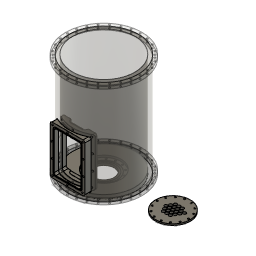
Smooth.SAQ.Pix.Vessel.5.9.2023. (Autodesk Fusion 360 design; units mm, degrees)
Autodesk Fusion 360 part; units mm, degrees
note: some values were not read from the file. Chosen so that the rebuilt part matches the saved one: which bodies a step acts on. Set by a fixed rule: which sketch regions a step uses.
sketch "Vessel.Base" plane through (0, 0, 0) normal (0, 1, 0) x (1, 0, 0)
  circle A0 centre (0, 0) radius 40
  circle A1 centre (0, 0) radius 30
  circle A2 centre (0, 0) radius 100
  circle A3 centre (0, 0) radius 110
  line L0 (0, 0) -> (105, 0) construction
  circle A4 centre (105, 0) radius 2.3
  circle A5 centre (102.3674, 23.3647) radius 2.3
  circle A6 centre (94.6017, 45.5578) radius 2.3
  circle A7 centre (82.0923, 65.4664) radius 2.3
  circle A8 centre (65.4664, 82.0923) radius 2.3
  circle A9 centre (45.5578, 94.6017) radius 2.3
  circle A10 centre (23.3647, 102.3674) radius 2.3
  circle A11 centre (0, 105) radius 2.3
  circle A12 centre (-23.3647, 102.3674) radius 2.3
  circle A13 centre (-45.5578, 94.6017) radius 2.3
  circle A14 centre (-65.4664, 82.0923) radius 2.3
  circle A15 centre (-82.0923, 65.4664) radius 2.3
  circle A16 centre (-94.6017, 45.5578) radius 2.3
  circle A17 centre (-102.3674, 23.3647) radius 2.3
  circle A18 centre (-105, 0) radius 2.3
  circle A19 centre (-102.3674, -23.3647) radius 2.3
  circle A20 centre (-94.6017, -45.5578) radius 2.3
  circle A21 centre (-82.0923, -65.4664) radius 2.3
  circle A22 centre (-65.4664, -82.0923) radius 2.3
  circle A23 centre (-45.5578, -94.6017) radius 2.3
  circle A24 centre (-23.3647, -102.3674) radius 2.3
  circle A25 centre (0, -105) radius 2.3
  circle A26 centre (23.3647, -102.3674) radius 2.3
  circle A27 centre (45.5578, -94.6017) radius 2.3
  circle A28 centre (65.4664, -82.0923) radius 2.3
  circle A29 centre (82.0923, -65.4664) radius 2.3
  circle A30 centre (94.6017, -45.5578) radius 2.3
  circle A31 centre (102.3674, -23.3647) radius 2.3
  circle A32 centre (0, 0) radius 90
  circle A33 centre (0, 0) radius 50
  line L1 (0, 0) -> (45, 0) construction
  circle A34 centre (45, 0) radius 2.3
  circle A35 centre (40.5436, 19.5248) radius 2.3
  circle A36 centre (28.057, 35.1824) radius 2.3
  circle A37 centre (10.0134, 43.8718) radius 2.3
  circle A38 centre (-10.0134, 43.8718) radius 2.3
  circle A39 centre (-28.057, 35.1824) radius 2.3
  circle A40 centre (-40.5436, 19.5248) radius 2.3
  circle A41 centre (-45, 0) radius 2.3
  circle A42 centre (-40.5436, -19.5248) radius 2.3
  circle A43 centre (-28.057, -35.1824) radius 2.3
  circle A44 centre (-10.0134, -43.8718) radius 2.3
  circle A45 centre (10.0134, -43.8718) radius 2.3
  circle A46 centre (28.057, -35.1824) radius 2.3
  circle A47 centre (40.5436, -19.5248) radius 2.3
  circle A48 centre (0, 0) radius 35
  line L2 (0, 0) -> (0, -105) construction
  line L3 (0, 0) -> (0, -95) construction
  dimension "d1" = 80
  dimension "d2" = 60
  dimension "d3" = 200
  dimension "d4" = 220
  dimension "d5" = 4.6
  dimension "d7" = 360
  dimension "d10" = 180
  dimension "d85" = 100
  dimension "d105" = 45
  dimension "d106" = 4.6
  dimension "d108" = 360
  dimension "d111" = 70
  dimension "d187" = 105
  dimension "d188" = 95
  constraint coincident A0.centre A1.centre
  constraint concentric A1 A2
  constraint concentric A2 A3
  constraint horizontal L0
  constraint coincident L0.end A4.centre
  constraint concentric A0 A33
  constraint horizontal L1
  constraint coincident L1.end A34.centre
  constraint concentric A33 A48
  constraint vertical L2
  constraint parallel L2 L3
  measures "d1" diameter of A0
  measures "d2" diameter of A1
  measures "d3" diameter of A2
  measures "d4" diameter of A3
  measures "d5" diameter of A4
  measures "d10" diameter of A32
  measures "d85" diameter of A33
  measures "d105" distance of A0.centre L1.end
  measures "d106" diameter of A34
  measures "d111" diameter of A48
  measures "d187" distance of A0.centre A25.centre
  measures "d188" distance of A0.centre L3.end
extrude "Extrude1" add sketch "Vessel.Base" along normal blind 10 contours A3 makes body 1
extrude "Extrude2" add sketch "Vessel.Base" along normal blind 300 separate body contours A2 makes body 2
extrude "Extrude3" add 1 faces at (-98.8073, 10, -35.1548) along direction (0, 1, 0) blind 10 separate body on bodies 1 makes body 3
move_body "Move1" bodies 3 to x (1, 0, 0) y (0, 1, 0) z (0, 0, 1) at (0, 280, 0)
extrude "Extrude5" add sketch "Vessel.Base" along normal blind 10 separate body contours A0 | A48 makes body 4
extrude "Extrude6" add sketch "Vessel.Base" along normal blind 11.6 contours A32 | A33 | A34 | A35 | A36 | A37 | A38 | A39 | A40 | A41 | A42 | A43 | A44 | A45 | A46 | A47 bodies 4
extrude "Extrude7" cut 1 faces at (36.4061, 10, 3.4777) along direction (0, -1, 0) blind 1.6 on bodies 4 bodies 4
sketch "Readout-Holder" plane through (0, 0, 0) normal (0, 1, 0) x (1, 0, 0)
  circle A0 centre (200, 0) radius 30
  circle A1 centre (200, 0) radius 1 construction
  circle A2 centre (210, 0) radius 1 construction
  circle A3 centre (220, 0) radius 1 construction
  circle A4 centre (180, 0) radius 1 construction
  circle A5 centre (205, 8.6603) radius 1 construction
  circle A6 centre (195, 8.6603) radius 1 construction
  circle A7 centre (190, 0) radius 1 construction
  circle A8 centre (195, -8.6603) radius 1 construction
  circle A9 centre (205, -8.6603) radius 1 construction
  circle A10 centre (210, 17.3205) radius 1 construction
  circle A11 centre (190, 17.3205) radius 1 construction
  circle A12 centre (180, 0) radius 1 construction
  circle A13 centre (190, -17.3205) radius 1 construction
  circle A14 centre (210, -17.3205) radius 1 construction
  circle A15 centre (200, 17.3205) radius 1 construction
  circle A16 centre (200, -17.3205) radius 1 construction
  circle A17 centre (185, 8.6603) radius 1 construction
  circle A18 centre (215, 8.6603) radius 1 construction
  circle A19 centre (185, -8.6603) radius 1 construction
  circle A20 centre (215, -8.6603) radius 1 construction
  circle A21 centre (200, 0) radius 40 construction
  circle A22 centre (200, 0) radius 4.5
  circle A23 centre (210, 0) radius 4.5
  circle A24 centre (220, 0) radius 4.5
  circle A25 centre (215, 8.6603) radius 4.5
  circle A26 centre (205, 8.6603) radius 4.5
  circle A27 centre (195, 8.6603) radius 4.5
  circle A28 centre (185, 8.6603) radius 4.5
  circle A29 centre (190, 17.3205) radius 4.5
  circle A30 centre (200, 17.3205) radius 4.5
  circle A31 centre (210, 17.3205) radius 4.5
  circle A32 centre (190, 0) radius 4.5
  circle A33 centre (180, 0) radius 4.5
  circle A34 centre (185, -8.6603) radius 4.5
  circle A35 centre (195, -8.6603) radius 4.5
  circle A36 centre (205, -8.6603) radius 4.5
  circle A37 centre (215, -8.6603) radius 4.5
  circle A38 centre (190, -17.3205) radius 4.5
  circle A39 centre (200, -17.3205) radius 4.5
  circle A40 centre (210, -17.3205) radius 4.5
  circle A41 centre (200, 0) radius 50
  line L0 (200, 0) -> (245, 0) construction
  circle A42 centre (245, 0) radius 2.3
  circle A43 centre (240.5436, 19.5248) radius 2.3
  circle A44 centre (228.057, 35.1824) radius 2.3
  circle A45 centre (210.0134, 43.8718) radius 2.3
  circle A46 centre (189.9866, 43.8718) radius 2.3
  circle A47 centre (171.943, 35.1824) radius 2.3
  circle A48 centre (159.4564, 19.5248) radius 2.3
  circle A49 centre (155, 0) radius 2.3
  circle A50 centre (159.4564, -19.5248) radius 2.3
  circle A51 centre (171.943, -35.1824) radius 2.3
  circle A52 centre (189.9866, -43.8718) radius 2.3
  circle A53 centre (210.0134, -43.8718) radius 2.3
  circle A54 centre (228.057, -35.1824) radius 2.3
  circle A55 centre (240.5436, -19.5248) radius 2.3
  line L1 (215, 8.6603) -> (225, 8.6603) construction
  circle A56 centre (225, 8.6603) radius 1 construction
  circle A57 centre (225, 8.6603) radius 4.5
  dimension "d23" = 60
  dimension "d25" = 2
  dimension "d28" = 20
  dimension "d29" = 0
  dimension "d32" = -20
  dimension "d33" = 0
  dimension "d35" = 360
  dimension "d37" = 360
  dimension "d39" = 2
  dimension "d41" = 2
  dimension "d46" = 2
  dimension "d47" = 2
  dimension "d48" = 2
  dimension "d49" = 2
  dimension "d52" = 80
  dimension "d63" = 9
  dimension "d64" = 9
  dimension "d65" = 9
  dimension "d66" = 9
  dimension "d67" = 9
  dimension "d68" = 9
  dimension "d69" = 9
  dimension "d70" = 9
  dimension "d71" = 9
  dimension "d72" = 9
  dimension "d73" = 9
  dimension "d74" = 9
  dimension "d75" = 9
  dimension "d76" = 9
  dimension "d77" = 9
  dimension "d78" = 9
  dimension "d79" = 9
  dimension "d80" = 9
  dimension "d100" = 4.6
  dimension "d102" = 360
  dimension "d117" = 10
  dimension "d118" = 2
  dimension "d119" = 9
  constraint concentric A0 A1
  constraint concentric A0 A21
  constraint concentric A1 A22
  constraint concentric A2 A23
  constraint concentric A3 A24
  constraint concentric A18 A25
  constraint concentric A5 A26
  constraint concentric A6 A27
  constraint concentric A17 A28
  constraint concentric A11 A29
  constraint concentric A15 A30
  constraint concentric A10 A31
  constraint concentric A7 A32
  constraint concentric A12 A33
  constraint concentric A19 A34
  constraint concentric A8 A35
  constraint concentric A9 A36
  constraint concentric A20 A37
  constraint concentric A13 A38
  constraint concentric A16 A39
  constraint concentric A14 A40
  constraint concentric A22 A41
  constraint coincident A0.centre A1.centre
  constraint horizontal L0
  constraint coincident L0.end A42.centre
  constraint horizontal L1
  constraint coincident A18.centre A25.centre
  constraint coincident L1.end A56.centre
  constraint concentric A56 A57
  measures "d23" diameter of A0
  measures "d25" diameter of A1
  measures "d39" diameter of A15
  measures "d41" diameter of A16
  measures "d46" diameter of A17
  measures "d47" diameter of A18
  measures "d48" diameter of A19
  measures "d49" diameter of A20
  measures "d52" diameter of A21
  measures "d63" diameter of A23
  measures "d64" diameter of A24
  measures "d65" diameter of A25
  measures "d66" diameter of A26
  measures "d67" diameter of A27
  measures "d68" diameter of A28
  measures "d69" diameter of A29
  measures "d70" diameter of A30
  measures "d71" diameter of A31
  measures "d72" diameter of A32
  measures "d73" diameter of A33
  measures "d74" diameter of A34
  measures "d75" diameter of A35
  measures "d76" diameter of A36
  measures "d77" diameter of A37
  measures "d78" diameter of A38
  measures "d79" diameter of A39
  measures "d80" diameter of A40
  measures "d100" diameter of A42
  measures "d117" distance of A18.centre L1.end
  measures "d118" diameter of A56
  measures "d119" diameter of A57
extrude "Extrude16" cut sketch "Vessel.Base" along normal blind 18 contours A1 bodies 4
extrude "Extrude17" cut sketch "Vessel.Base" along normal blind 14 contours A0 | A33 | A34 | A35 | A36 | A37 | A38 | A39 | A40 | A41 | A42 | A43 | A44 | A45 | A46 | A47 | A48 bodies 4
extrude "Extrude18" add sketch "Vessel.Base" along normal blind 2 contours A0 | A33 | A34 | A35 | A36 | A37 | A38 | A39 | A40 | A41 | A42 | A43 | A44 | A45 | A46 | A47 | A48 bodies 4
extrude "Extrude19" add 1 faces at (43.0355, 2, 3.9745) along direction (0, 1, 0) blind 4 on bodies 4 bodies 4
extrude "Extrude20" add sketch "Readout-Holder" along normal blind 8 separate body contours A0 A57 | A41 | A42 | A43 | A44 | A45 | A46 | A47 | A48 | A49 | A50 | A51 | A52 | A53 | A54 | A55 picked at (228.6545, 9.8725) makes body 5
extrude "Extrude21" cut sketch "Readout-Holder" along normal blind 4 contours A0 A57 | A41 | A42 | A43 | A44 | A45 | A46 | A47 | A48 | A49 | A50 | A51 | A52 | A53 | A54 | A55 picked at (228.6545, 9.8725) bodies 5
extrude "Extrude22" add sketch "Readout-Holder" along normal blind 8 contours A0 A57 | A0 A57 picked at (176.7568, 7.7937) picked at (225.7718, 9.0442) bodies 5
extrude "Extrude23" cut sketch "Readout-Holder" along normal blind 20 contours A42 | A43 | A44 | A45 | A46 | A47 | A48 | A49 | A50 | A51 | A52 | A53 | A54 | A55 bodies 5
extrude "Extrude24" cut sketch "Vessel.Base" along normal blind 24 contours A34 | A35 | A36 | A37 | A38 | A39 | A40 | A41 | A42 | A43 | A44 | A45 | A46 | A47 bodies 4
extrude "Extrude25" cut sketch "Vessel.Base" along normal blind 1 from surface at 5 contours A0 bodies 4
sketch "Door.Hole" plane through (0, 0, 0) normal (0, 0, 1) x (1, 0, 0)
  line L0 (-35, 30) -> (35, 30)
  line L1 (40, 35) -> (40, 145)
  line L2 (35, 150) -> (-35, 150)
  line L3 (-40, 145) -> (-40, 35)
  line L4 (-45, 20) -> (45, 20)
  line L5 (50, 25) -> (50, 155)
  line L6 (45, 160) -> (-45, 160)
  line L7 (-50, 155) -> (-50, 25)
  circle A0 centre (0, 155) radius 2.3
  circle A1 centre (45, 155) radius 2.3 construction
  circle A2 centre (-45, 111.6667) radius 2.3
  circle A3 centre (45, 111.6667) radius 2.3
  circle A4 centre (-45, 68.3333) radius 2.3
  circle A5 centre (45, 68.3333) radius 2.3
  circle A6 centre (0, 25) radius 2.3
  arc A7 (-35, 150) -> (-40, 145) centre (-35, 145) ccw
  arc A8 (40, 145) -> (35, 150) centre (35, 145) ccw
  arc A9 (-40, 35) -> (-35, 30) centre (-35, 35) ccw
  arc A10 (35, 30) -> (40, 35) centre (35, 35) ccw
  arc A11 (-45, 160) -> (-50, 155) centre (-45, 155) ccw
  arc A12 (50, 155) -> (45, 160) centre (45, 155) ccw
  arc A13 (45, 20) -> (50, 25) centre (45, 25) ccw
  arc A14 (-50, 25) -> (-45, 20) centre (-45, 25) ccw
  line L8 (-35, 155) -> (35, 155) construction
  line L9 (45, 145) -> (45, 35) construction
  line L10 (35, 25) -> (-35, 25) construction
  line L11 (-45, 35) -> (-45, 145) construction
  arc A15 (-35, 155) -> (-45, 145) centre (-35, 145) ccw construction
  arc A16 (45, 145) -> (35, 155) centre (35, 145) ccw construction
  arc A17 (35, 25) -> (45, 35) centre (35, 35) ccw construction
  arc A18 (-45, 35) -> (-35, 25) centre (-35, 35) ccw construction
  line L12 (-34.5711, 152.0711) -> (34.5711, 152.0711)
  line L13 (42.0711, 144.5711) -> (42.0711, 35.4289)
  line L14 (34.5711, 27.9289) -> (-34.5711, 27.9289)
  line L15 (-42.0711, 35.4289) -> (-42.0711, 144.5711)
  arc A19 (-34.5711, 152.0711) -> (-42.0711, 144.5711) centre (-34.5711, 144.5711) ccw
  arc A20 (42.0711, 144.5711) -> (34.5711, 152.0711) centre (34.5711, 144.5711) ccw
  arc A21 (34.5711, 27.9289) -> (42.0711, 35.4289) centre (34.5711, 35.4289) ccw
  arc A22 (-42.0711, 35.4289) -> (-34.5711, 27.9289) centre (-34.5711, 35.4289) ccw
  line L16 (-33.5355, 148.5355) -> (33.5355, 148.5355)
  line L17 (38.5355, 143.5355) -> (38.5355, 36.4645)
  line L18 (33.5355, 31.4645) -> (-33.5355, 31.4645)
  line L19 (-38.5355, 36.4645) -> (-38.5355, 143.5355)
  arc A23 (-33.5355, 148.5355) -> (-38.5355, 143.5355) centre (-33.5355, 143.5355) ccw
  arc A24 (38.5355, 143.5355) -> (33.5355, 148.5355) centre (33.5355, 143.5355) ccw
  arc A25 (33.5355, 31.4645) -> (38.5355, 36.4645) centre (33.5355, 36.4645) ccw
  arc A26 (-38.5355, 36.4645) -> (-33.5355, 31.4645) centre (-33.5355, 36.4645) ccw
  line L20 (-45, 25) -> (-42.0711, 27.9289) construction
  circle A27 centre (-43.3737, 26.6263) radius 2.3
  line L21 (-45, 155) -> (-39.8744, 149.8744) construction
  line L22 (45, 155) -> (39.8744, 149.8744) construction
  line L23 (45, 25) -> (39.8744, 30.1256) construction
  circle A28 centre (43.3737, 26.6263) radius 2.3
  circle A29 centre (-43.3737, 153.3737) radius 2.3
  circle A30 centre (43.3737, 153.3737) radius 2.3
  circle A31 centre (-45, 155) radius 2.3 construction
  circle A32 centre (-45, 25) radius 2.3 construction
  circle A33 centre (45, 25) radius 2.3 construction
  point P0 (-40, 30)
  point P1 (40, 30)
  point P2 (-40, 150)
  point P3 (-50, 20)
  point P4 (50, 20)
  point P5 (-50, 160)
  dimension "d143" = 80
  dimension "d144" = 120
  dimension "d147" = 100
  dimension "d148" = 140
  dimension "d154" = 5
  dimension "d155" = 5
  dimension "d156" = 5
  dimension "d157" = 5
  dimension "d158" = 5
  dimension "d159" = 5
  dimension "d160" = 5
  dimension "d161" = 5
  dimension "d162" = 10
  dimension "d163" = 10
  dimension "d164" = 10
  dimension "d165" = 10
  dimension "d166" = 7.5
  dimension "d167" = 7.5
  dimension "d168" = 7.5
  dimension "d169" = 7.5
  dimension "d170" = 5
  dimension "d171" = 5
  dimension "d172" = 5
  dimension "d173" = 5
  dimension "d174" = 4.6
  dimension "d175" = 4.6
  dimension "d176" = 4.6
  dimension "d177" = 4.6
  dimension "d178" = 4.6
  dimension "d179" = 4.6
  dimension "d180" = 4.6
  constraint horizontal L0
  constraint vertical L1
  constraint horizontal L2
  constraint vertical L3
  constraint horizontal L4
  constraint vertical L5
  constraint horizontal L6
  constraint vertical L7
  constraint coincident P2 L3
  constraint coincident P2 L2
  constraint tangent L3 A7
  constraint tangent L2 A7
  constraint tangent L2 A8
  constraint tangent L1 A8
  constraint coincident P0 L3
  constraint coincident P0 L0
  constraint tangent L3 A9
  constraint tangent L0 A9
  constraint coincident P1 L0
  constraint coincident P1 L1
  constraint tangent L0 A10
  constraint tangent L1 A10
  constraint coincident P5 L7
  constraint coincident P5 L6
  constraint tangent L7 A11
  constraint tangent L6 A11
  constraint tangent L6 A12
  constraint tangent L5 A12
  constraint coincident P4 L4
  constraint coincident P4 L5
  constraint tangent L4 A13
  constraint tangent L5 A13
  constraint coincident P3 L7
  constraint coincident P3 L4
  constraint tangent L7 A14
  constraint tangent L4 A14
  constraint horizontal L8
  constraint vertical L9
  constraint horizontal L10
  constraint vertical L11
  constraint tangent L11 A15
  constraint tangent L8 A15
  constraint tangent L8 A16
  constraint tangent L9 A16
  constraint tangent L10 A17
  constraint tangent L9 A17
  constraint tangent L10 A18
  constraint tangent L11 A18
  constraint horizontal L12
  constraint vertical L13
  constraint horizontal L14
  constraint vertical L15
  constraint tangent L15 A19
  constraint tangent L12 A19
  constraint tangent L12 A20
  constraint tangent L13 A20
  constraint tangent L14 A21
  constraint tangent L13 A21
  constraint tangent L15 A22
  constraint tangent L14 A22
  constraint horizontal L16
  constraint vertical L17
  constraint horizontal L18
  constraint vertical L19
  constraint tangent L19 A23
  constraint tangent L16 A23
  constraint tangent L16 A24
  constraint tangent L17 A24
  constraint tangent L17 A25
  constraint tangent L18 A25
  constraint tangent L19 A26
  constraint tangent L18 A26
  constraint midpoint A18 L20.end
  constraint coincident L20 A27.centre
  constraint coincident A11.centre L21.start
  constraint midpoint A19 L21.end
  constraint coincident A1.centre A12.centre
  constraint midpoint A20 L22.end
  constraint coincident A13.centre L23.start
  constraint midpoint A21 L23.end
  constraint coincident L23 A28.centre
  constraint coincident L21 A29.centre
  constraint coincident A1 A30.centre
  constraint coincident L22 A30.centre
  constraint concentric A11 A31
  constraint coincident A14.centre L20.start
  measures "d143" distance of P0 P1
  measures "d144" distance of P0 P2
  measures "d147" distance of P3 P4
  measures "d148" distance of P3 P5
  measures "d154" radius of A7
  measures "d155" radius of A8
  measures "d156" radius of A9
  measures "d157" radius of A10
  measures "d158" radius of A11
  measures "d159" radius of A12
  measures "d160" radius of A13
  measures "d161" radius of A14
  measures "d162" radius of A15
  measures "d163" radius of A16
  measures "d164" radius of A17
  measures "d165" radius of A18
  measures "d166" radius of A19
  measures "d167" radius of A20
  measures "d168" radius of A21
  measures "d169" radius of A22
  measures "d170" radius of A23
  measures "d171" radius of A24
  measures "d172" radius of A25
  measures "d173" radius of A26
  measures "d174" diameter of A27
  measures "d175" diameter of A28
  measures "d176" diameter of A29
  measures "d177" diameter of A30
  measures "d178" diameter of A31
  measures "d179" diameter of A32
  measures "d180" diameter of A33
extrude "Extrude26" cut sketch "Readout-Holder" along normal blind 9 contours A0 A57 | A0 A57 picked at (225.7718, 9.0442) picked at (228.6545, 9.8725) bodies 5
extrude "Extrude28" add 1 faces at (172.0133, 8, -21.645) along direction (0, 1, 0) blind 6 on bodies 5 bodies 5
extrude "Extrude29" cut 1 faces at (237.6454, 4, 8.4486) along direction (0, 1, 0) blind 2 on bodies 5 bodies 5
extrude "Extrude30" cut 1 faces at (172.0133, 14, -21.645) along direction (0, -1, 0) blind 2 on bodies 5 bodies 5
extrude "Extrude31" cut 1 faces at (172.0133, 12, -21.645) along direction (0, -1, 0) blind 2 on bodies 5 bodies 5
extrude "Extrude35" add sketch "Door.Hole" along normal blind 10 and the other way blind 25 from surface at 95 separate body makes body 6 at (-40, 108.3333, 93.3333) makes body 7 at (-50, 111.6667, 81.6667)
extrude "Extrude36" cut sketch "Vessel.Base" along normal blind 180 contours A2 bodies 6 7 makes body 9 at (-29.4946, 25.286, 95.5514) makes body 8 at (-40, 108.3333, 96.101)
extrude "Extrude37" cut sketch "Door.Hole" along normal blind 180 contours L16 L17 L18 L19 A23 A24 A25 A26 bodies 2
sketch "Inner.Door.Cleaner" plane through (0, 0, 0) normal (0, 1, 0) x (1, 0, 0)
  circle A0 centre (0, 0) radius 85 construction
  line L0 (0, 0) -> (0, -80) construction
  line L1 (0, -80) -> (25, -80) construction
  line L2 (25, -80) -> (25, -70) construction
  line L3 (25, -70) -> (0, -70) construction
  line L4 (0, -70) -> (0, -80) construction
  line L5 (25, -70) -> (-25, -70)
  line L6 (-25, -70) -> (-25, -70)
  line L7 (-15, -80) -> (15, -80)
  line L8 (25, -70) -> (25, -70)
  arc A1 (-25, -70) -> (-15, -80) centre (-15, -70) ccw
  arc A2 (15, -80) -> (25, -70) centre (15, -70) ccw
  point P0 (14.7189, -80)
  dimension "d198" = 170
  dimension "d199" = 80
  dimension "d200" = 25
  dimension "d201" = 10
  dimension "d202" = 50
  dimension "d203" = 10
  dimension "d204" = 10
  dimension "d205" = 10
  constraint coincident A0.centre L0.start
  constraint vertical L0
  constraint horizontal L1
  constraint vertical L2
  constraint horizontal L3
  constraint vertical L4
  constraint horizontal L5
  constraint horizontal L7
  constraint tangent L7 A1
  constraint coincident P0 L8
  constraint coincident P0 L7
  constraint tangent L7 A2
  measures "d198" diameter of A0
  measures "d199" distance of A0.centre L0.end
  measures "d200" distance of L0.end L1.end
  measures "d201" distance of L0.end L3.end
  measures "d202" distance of L2.end L5.end
  measures "d203" distance of L2.end P0
  measures "d204" radius of A1
  measures "d205" radius of A2
extrude "Extrude38" cut sketch "Inner.Door.Cleaner" along normal blind 175 bodies 6 7
extrude "Extrude39" cut sketch "Door.Hole" along normal blind 130 contours A0 | A2 | A3 | A4 | A5 | A6 | A27 | A28 | A29 | A30 bodies 2
extrude "Extrude40" add sketch "Door.Hole" along normal blind 35 from surface at 70 separate body contours L12 L13 L14 L15 A19 A20 A21 A22 makes body 10
extrude "Extrude41" cut sketch "Vessel.Base" along normal blind 180 contours A2 bodies 10 makes body 11 at (-42.0711, 71.8096, 95.4797)
sketch "Sketch6" plane through (0, 0, 0) normal (0, 1, 0) x (1, 0, 0)
  circle A0 centre (0, 0) radius 100
  circle A1 centre (0, 0) radius 101
  circle A2 centre (0, 0) radius 90
  circle A3 centre (0, 0) radius 89
  dimension "d216" = 200
  dimension "d217" = 202
  dimension "d218" = 180
  dimension "d219" = 178
  constraint coincident A0.centre A1.centre
  constraint concentric A0 A1
  constraint concentric A1 A2
  constraint concentric A2 A3
  measures "d216" diameter of A0
  measures "d217" diameter of A1
  measures "d218" diameter of A2
  measures "d219" diameter of A3
extrude "Extrude42" cut sketch "Sketch6" along normal blind 155 bodies 10 11
extrude "Extrude32" [suppressed]
extrude "Extrude27" [suppressed]
extrude "Extrude8" [suppressed]
extrude "Extrude10" [suppressed]
extrude "Extrude11" [suppressed]
extrude "Extrude12" [suppressed]
extrude "Extrude13" [suppressed]
extrude "Extrude14" [suppressed]
extrude "Extrude15" [suppressed]
extrude "Extrude9" [suppressed]
extrude "Extrude4" [suppressed]
named bodies: "Ring.1", "Cylinder.Wall", "Ring.2", "Vessel.Base", "Readout.Support"
